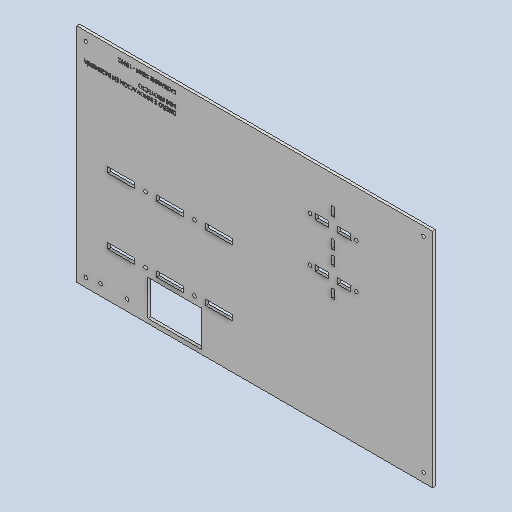
# Autodesk Inventor part: Base_proyecto
Saved by Autodesk Inventor 2022 (Build 260153000, 153)
## iProperties
Created: 2022-02-22
Part Number: Base_proyecto
Material: Generic
Document SubType Name: Modeling
Designer: katha
Density: 1 g/cm^3
Appearance: Default
Author: katha
Autodesk Inventor part; units mm, degrees
(part 1 of 2)
ref_plane "YZ Plane" through (0, 0, 0) normal (1, 0, 0) x (0, 1, 0)
ref_plane "XZ Plane" through (0, 0, 0) normal (0, 1, 0) x (-1, 0, 0)
ref_plane "XY Plane" through (0, 0, 0) normal (0, 0, 1) x (1, 0, 0)
sketch "Sketch1" plane through (0, 0, 0) normal (0, 0, 1) x (1, 0, 0)
  line L0 (200, 125) -> (-200, 125)
  line L1 (-200, 125) -> (-200, -125)
  line L2 (-200, -125) -> (200, -125)
  line L3 (200, -125) -> (200, 125)
  line L4 (200, 125) -> (-200, -125) construction
  line L5 (-200, 125) -> (200, -125) construction
  point P0 (0, 0)
  dimension "d0" = 400
  dimension "d1" = 250
  constraints: 12 end point, 2 midpoint, 2 parallel, 1 horizontal, 1 perpendicular
  measures "d0" distance of L2.end L1.end
  measures "d1" distance of L1.end L0.end
extrude "Extrusion1" add sketch "Sketch1" along normal blind 3.2
sketch "Sketch2" plane through (0, 0, 0) normal (0, 0, -1) x (-1, 0, 0)
  line L0 (-116.4, 20) -> (-116.4, 26.2) projected
  line L1 (-112.4, 26.2) -> (-112.4, 20) projected
  line L2 (-64.4, 20) -> (-64.4, 26.2) projected
  line L3 (-60.4, 26.2) -> (-60.4, 20) projected
  line L4 (-116.4, 70.2) -> (-116.4, 76.4) projected
  line L5 (-112.4, 76.4) -> (-112.4, 70.2) projected
  line L6 (-64.4, 70.2) -> (-64.4, 76.4) projected
  line L7 (-60.4, 76.4) -> (-60.4, 70.2) projected
  line L8 (-93.4, 76.4) -> (-108.4, 76.4) projected
  line L9 (-93.4, 70.2) -> (-108.4, 70.2) projected
  line L10 (-93.4, 76.4) -> (-93.4, 70.2) projected
  line L11 (-108.4, 76.4) -> (-108.4, 70.2) projected
  line L12 (-68.4, 76.4) -> (-83.4, 76.4) projected
  line L13 (-68.4, 70.2) -> (-83.4, 70.2) projected
  line L14 (-68.4, 76.4) -> (-68.4, 70.2) projected
  line L15 (-83.4, 76.4) -> (-83.4, 70.2) projected
  line L16 (-93.4, 26.2) -> (-108.4, 26.2) projected
  line L17 (-93.4, 20) -> (-108.4, 20) projected
  line L18 (-93.4, 26.2) -> (-93.4, 20) projected
  line L19 (-108.4, 26.2) -> (-108.4, 20) projected
  line L20 (-68.4, 26.2) -> (-83.4, 26.2) projected
  line L21 (-68.4, 20) -> (-83.4, 20) projected
  line L22 (-68.4, 26.2) -> (-68.4, 20) projected
  line L23 (-83.4, 26.2) -> (-83.4, 20) projected
  line L24 (69.5467, 5.2) -> (69.5467, -1) projected
  line L25 (25, 5.2) -> (55, 5.2) projected
  line L26 (80.0934, 5.2) -> (110.0934, 5.2) projected
  line L27 (124.6401, 5.2) -> (124.6401, -1) projected
  line L28 (135.1868, 5.2) -> (165.1868, 5.2) projected
  line L29 (55, -75) -> (25, -75) projected
  line L30 (110.0934, -75) -> (80.0934, -75) projected
  line L31 (165.1868, -75) -> (135.1868, -75) projected
  line L32 (124.6401, -68.8) -> (124.6401, -75) projected
  line L33 (69.5467, -68.8) -> (69.5467, -75) projected
  line L34 (-90, 35.2) -> (-90, 45.2) projected
  line L35 (-86.8, 45.2) -> (-86.8, 35.2) projected
  line L36 (-90, 35.2) -> (-86.8, 35.2) projected
  line L37 (-90, 45.2) -> (-86.8, 45.2) projected
  line L38 (-90, 51.2) -> (-86.8, 51.2) projected
  line L39 (-90, 51.2) -> (-90, 61.2) projected
  line L40 (-86.8, 61.2) -> (-86.8, 51.2) projected
  line L41 (-90, 61.2) -> (-86.8, 61.2) projected
  line L42 (165.1868, -1) -> (165.1868, 5.2) projected
  line L43 (165.1868, -1) -> (135.1868, -1) projected
  line L44 (135.1868, -1) -> (135.1868, 5.2) projected
  line L45 (120.6401, -1) -> (120.6401, 5.2) projected
  line L46 (124.6401, 5.2) -> (124.6401, -1) projected
  line L47 (65.5467, -1) -> (65.5467, 5.2) projected
  line L48 (120.6401, -75) -> (120.6401, -68.8) projected
  line L49 (135.1868, -75) -> (135.1868, -68.8) projected
  line L50 (135.1868, -68.8) -> (165.1868, -68.8) projected
  line L51 (165.1868, -75) -> (165.1868, -68.8) projected
  line L52 (80.0934, -68.8) -> (110.0934, -68.8) projected
  line L53 (80.0934, -75) -> (80.0934, -68.8) projected
  line L54 (110.0934, -75) -> (110.0934, -68.8) projected
  line L55 (25, -75) -> (25, -68.8) projected
  line L56 (25, -68.8) -> (55, -68.8) projected
  line L57 (55, -75) -> (55, -68.8) projected
  line L58 (65.5467, -75) -> (65.5467, -68.8) projected
  line L59 (55, -1) -> (25, -1) projected
  line L60 (25, -1) -> (25, 5.2) projected
  line L61 (55, -1) -> (55, 5.2) projected
  line L62 (80.0934, -1) -> (80.0934, 5.2) projected
  line L63 (110.0934, -1) -> (80.0934, -1) projected
  line L64 (110.0934, -1) -> (110.0934, 5.2) projected
  line L65 (55, -71.9) -> (135.1868, -71.9) construction
  line L66 (55, 2.1) -> (135.1868, 2.1) construction
  line L67 (64.0467, -68.8) -> (71.0467, -68.8) projected
  circle A0 centre (67.5467, -71.9) radius 2
  line L68 (95.0934, -68.8) -> (95.0934, -1) construction
  line L69 (95.0934, -34.9) -> (76.0096, -34.9) construction
  line L70 (67.5467, -68.8) -> (67.5467, -71.9) construction
  circle A1 centre (122.6401, -71.9) radius 2
  circle A2 centre (67.5467, 2.1) radius 2
  circle A3 centre (122.6401, 2.1) radius 2
  line L71 (-116.4, 23.1) -> (-112.4, 23.1) construction
  line L72 (-88.4, 45.2) -> (-88.4, 51.2) construction
  line L73 (-88.4, 48.2) -> (-97.8436, 48.2) construction
  circle A4 centre (-114.4, 23.1) radius 2
  circle A5 centre (-62.4, 23.1) radius 2
  circle A6 centre (-114.4, 73.3) radius 2
  circle A7 centre (-62.4, 73.3) radius 2
  line L74 (-90, 3.2) -> (-86.8, 3.2) projected
  line L75 (-90, 3.2) -> (-90, 13.2) projected
  line L76 (-86.8, 13.2) -> (-86.8, 3.2) projected
  line L77 (-90, 13.2) -> (-86.8, 13.2) projected
  line L78 (-90, 93.2) -> (-86.8, 93.2) projected
  line L79 (-90, 83.2) -> (-90, 93.2) projected
  line L80 (-86.8, 93.2) -> (-86.8, 83.2) projected
  line L81 (-90, 83.2) -> (-86.8, 83.2) projected
  line L82 (200, 125) -> (200, -125) projected
  point P0 (0, 0)
  dimension "d4" = 4
  dimension "d5" = 4
  constraints: 16 end point, 14 midpoint, 8 centre point, 6 symmetric about line, 2 horizontal, 1 point on line, 1 vertical, 6 other
  measures "d4" diameter of A0
  measures "d5" diameter of A4
extrude "Extrusion2" cut sketch "Sketch2" against normal blind 10 contours L10 L9 L11 L8 | L14 L13 L15 L12 | L18 L17 L19 L16 | L22 L21 L23 L20 | L25 L61 L59 L60 | L26 L64 L63 L62 | L28 L42 L43 L44 | L29 L55 L56 L57 | L30 L53 L52 L54 | L31 L49 L50 L51 | A0 | L34 L37 L35 L36 | L39 L41 L40 L38 | A1 | A2 | A3 | A4 | A5 | A6 | A7 | L75 L77 L76 L74 | L78 L80 L81 L79
sketch "Sketch3" plane through (0, 0, 3.2) normal (0, 0, 1) x (1, 0, 0)
  line L0 (-88.1097, 91.9364) -> (-249.5972, 91.9364) construction
  line L1 (-249.5972, 91.9364) -> (-249.5972, 106.9237) construction
  line L2 (-249.5972, 106.9237) -> (-88.1097, 106.9237) construction
  line L3 (-88.1097, 106.9237) -> (-88.1097, 91.9364) construction
  line L4 (-88.5956, 97.0895) -> (-88.5956, 93.0895)
  line L5 (-88.5956, 93.0895) -> (-89.4247, 93.0895)
  spline S0 degree 2 poles (-89.4247, 93.0895) (-90.3219, 93.0895) (-90.7267, 93.232) knots 0 0 0 1 1 1
  spline S1 degree 2 poles (-90.7267, 93.232) (-91.3097, 93.436) (-91.964, 94.4433) (-91.964, 95.1397) knots 0 0 0 1 2 2 2
  spline S2 degree 2 poles (-91.964, 95.1397) (-91.964, 95.7421) (-91.4458, 96.6555) (-90.6166, 97.0895) (-89.8684, 97.0895) knots 0 0 0 1 2 3 3 3
  line L6 (-89.8684, 97.0895) -> (-88.5956, 97.0895)
  line L7 (-88.9778, 96.7105) -> (-89.4409, 96.7105)
  spline S3 degree 2 poles (-89.4409, 96.7105) (-90.2701, 96.7105) (-90.5907, 96.6069) knots 0 0 0 1 1 1
  spline S4 degree 2 poles (-90.5907, 96.6069) (-91.0409, 96.4611) (-91.5591, 95.6967) (-91.5591, 95.1461) knots 0 0 0 1 2 2 2
  spline S5 degree 2 poles (-91.5591, 95.1461) (-91.5591, 94.5664) (-90.9988, 93.7469) (-90.4968, 93.5947) knots 0 0 0 1 2 2 2
  spline S6 degree 2 poles (-90.4968, 93.5947) (-90.1243, 93.4814) (-89.2595, 93.4814) knots 0 0 0 1 1 1
  line L8 (-89.2595, 93.4814) -> (-88.9778, 93.4814)
  line L9 (-88.9778, 93.4814) -> (-88.9778, 96.7105)
  line L10 (-92.683, 93.0895) -> (-93.0814, 93.0895)
  line L11 (-93.0814, 93.0895) -> (-93.0814, 97.0895)
  line L12 (-93.0814, 97.0895) -> (-92.683, 97.0895)
  line L13 (-92.683, 97.0895) -> (-92.683, 93.0895)
  line L14 (-93.5867, 96.3445) -> (-93.9267, 96.1405)
  spline S7 degree 2 poles (-93.9267, 96.1405) (-94.2863, 96.8012) (-94.7559, 96.8012) knots 0 0 0 1 1 1
  spline S8 degree 2 poles (-94.7559, 96.8012) (-94.9567, 96.8012) (-95.3097, 96.6133) (-95.4944, 96.2992) (-95.4944, 96.121) knots 0 0 0 1 2 3 3 3
  spline S9 degree 2 poles (-95.4944, 96.121) (-95.4944, 95.9202) (-95.3583, 95.7291) knots 0 0 0 1 1 1
  spline S10 degree 2 poles (-95.3583, 95.7291) (-95.1705, 95.4603) (-94.6749, 95.0846) knots 0 0 0 1 1 1
  spline S11 degree 2 poles (-94.6749, 95.0846) (-94.1729, 94.7089) (-94.0498, 94.5405) knots 0 0 0 1 1 1
  spline S12 degree 2 poles (-94.0498, 94.5405) (-93.8393, 94.2555) (-93.8393, 93.9283) knots 0 0 0 1 1 1
  spline S13 degree 2 poles (-93.8393, 93.9283) (-93.8393, 93.666) (-94.0887, 93.2352) (-94.5421, 92.9891) (-94.8077, 92.9891) knots 0 0 0 1 2 3 3 3
  spline S14 degree 2 poles (-94.8077, 92.9891) (-95.0927, 92.9891) (-95.5818, 93.2708) (-95.8571, 93.6465) knots 0 0 0 1 2 2 2
  line L15 (-95.8571, 93.6465) -> (-95.53, 93.8927)
  spline S15 degree 2 poles (-95.53, 93.8927) (-95.3065, 93.5947) (-94.9858, 93.4036) (-94.8012, 93.4036) knots 0 0 0 1 2 2 2
  spline S16 degree 2 poles (-94.8012, 93.4036) (-94.5583, 93.4036) (-94.2506, 93.6984) (-94.2506, 93.9121) knots 0 0 0 1 2 2 2
  spline S17 degree 2 poles (-94.2506, 93.9121) (-94.2506, 94.0417) (-94.3607, 94.2878) (-94.5033, 94.4303) knots 0 0 0 1 2 2 2
  spline S18 degree 2 poles (-94.5033, 94.4303) (-94.581, 94.5081) (-95.0215, 94.832) knots 0 0 0 1 1 1
  spline S19 degree 2 poles (-95.0215, 94.832) (-95.5397, 95.2142) (-95.9251, 95.8133) (-95.9251, 96.1146) knots 0 0 0 1 2 2 2
  spline S20 degree 2 poles (-95.9251, 96.1146) (-95.9251, 96.5486) (-95.2644, 97.1899) (-94.7915, 97.1899) knots 0 0 0 1 2 2 2
  spline S21 degree 2 poles (-94.7915, 97.1899) (-94.4288, 97.1899) (-93.8361, 96.8012) (-93.5867, 96.3445) knots 0 0 0 1 2 2 2
  line L16 (-96.7737, 93.0895) -> (-99.0668, 93.0895)
  line L17 (-99.0668, 93.0895) -> (-99.0668, 93.4814)
  line L18 (-99.0668, 93.4814) -> (-97.1721, 93.4814)
  line L19 (-97.1721, 93.4814) -> (-97.1721, 94.7348)
  line L20 (-97.1721, 94.7348) -> (-99.0506, 94.7348)
  line L21 (-99.0506, 94.7348) -> (-99.0506, 95.1267)
  line L22 (-99.0506, 95.1267) -> (-97.1721, 95.1267)
  line L23 (-97.1721, 95.1267) -> (-97.1721, 96.6976)
  line L24 (-97.1721, 96.6976) -> (-99.0506, 96.6976)
  line L25 (-99.0506, 96.6976) -> (-99.0506, 97.0895)
  line L26 (-99.0506, 97.0895) -> (-96.7737, 97.0895)
  line L27 (-96.7737, 97.0895) -> (-96.7737, 93.0895)
  line L28 (-99.7599, 97.0895) -> (-99.7599, 93.0895)
  line L29 (-99.7599, 93.0895) -> (-99.8474, 93.0895)
  line L30 (-99.8474, 93.0895) -> (-102.5097, 96.1534)
  line L31 (-102.5097, 96.1534) -> (-102.5097, 93.0895)
  line L32 (-102.5097, 93.0895) -> (-102.9049, 93.0895)
  line L33 (-102.9049, 93.0895) -> (-102.9049, 97.0895)
  line L34 (-102.9049, 97.0895) -> (-102.8142, 97.0895)
  line L35 (-102.8142, 97.0895) -> (-100.1745, 94.0611)
  line L36 (-100.1745, 94.0611) -> (-100.1745, 97.0895)
  line L37 (-100.1745, 97.0895) -> (-99.7599, 97.0895)
  line L38 (-102.1373, 92.2247) -> (-102.3284, 92.487)
  spline S22 degree 2 poles (-102.3284, 92.487) (-102.134, 92.6295) (-101.8652, 92.7299) (-101.713, 92.7299) knots 0 0 0 1 2 2 2
  spline S23 degree 2 poles (-101.713, 92.7299) (-101.5186, 92.7299) (-101.3114, 92.6295) knots 0 0 0 1 1 1
  spline S24 degree 2 poles (-101.3114, 92.6295) (-101.1365, 92.5421) (-101.0879, 92.5291) knots 0 0 0 1 1 1
  spline S25 degree 2 poles (-101.0879, 92.5291) (-101.0199, 92.5097) (-100.9454, 92.5097) knots 0 0 0 1 1 1
  spline S26 degree 2 poles (-100.9454, 92.5097) (-100.8514, 92.5097) (-100.6798, 92.5777) (-100.5146, 92.6976) knots 0 0 0 1 2 2 2
  line L39 (-100.5146, 92.6976) -> (-100.3365, 92.419)
  spline S27 degree 2 poles (-100.3365, 92.419) (-100.5826, 92.1534) (-100.9486, 92.1534) knots 0 0 0 1 1 1
  spline S28 degree 2 poles (-100.9486, 92.1534) (-101.1203, 92.1534) (-101.3632, 92.2635) knots 0 0 0 1 1 1
  spline S29 degree 2 poles (-101.3632, 92.2635) (-101.5931, 92.3737) (-101.7292, 92.3737) knots 0 0 0 1 1 1
  spline S30 degree 2 poles (-101.7292, 92.3737) (-101.8782, 92.3737) (-102.1373, 92.2247) knots 0 0 0 1 1 1
  spline S31 degree 2 poles (-105.7842, 92.9891) (-106.6911, 92.9891) (-107.9154, 94.2004) (-107.9154, 95.0878) knots 0 0 0 1 2 2 2
  spline S32 degree 2 poles (-107.9154, 95.0878) (-107.9154, 95.9656) (-106.6944, 97.1899) (-105.8166, 97.1899) knots 0 0 0 1 2 2 2
  spline S33 degree 2 poles (-105.8166, 97.1899) (-104.9259, 97.1899) (-103.7016, 95.972) (-103.7016, 95.1073) knots 0 0 0 1 2 2 2
  spline S34 degree 2 poles (-103.7016, 95.1073) (-103.7016, 94.5308) (-104.2587, 93.5461) (-105.2239, 92.9891) (-105.7842, 92.9891) knots 0 0 0 1 2 3 3 3
  spline S35 degree 2 poles (-105.8004, 93.3777) (-105.3567, 93.3777) (-104.5599, 93.8409) (-104.113, 94.6247) (-104.113, 95.1073) knots 0 0 0 1 2 3 3 3
  spline S36 degree 2 poles (-104.113, 95.1073) (-104.113, 95.8198) (-105.1041, 96.8012) (-105.8004, 96.8012) knots 0 0 0 1 2 2 2
  spline S37 degree 2 poles (-105.8004, 96.8012) (-106.2668, 96.8012) (-107.0603, 96.351) (-107.5041, 95.5672) (-107.5041, 95.0878) knots 0 0 0 1 2 3 3 3
  spline S38 degree 2 poles (-107.5041, 95.0878) (-107.5041, 94.6117) (-107.0603, 93.8409) (-106.2539, 93.3777) (-105.8004, 93.3777) knots 0 0 0 1 2 3 3 3
  line L40 (-110.2603, 93.0895) -> (-112.5535, 93.0895)
  line L41 (-112.5535, 93.0895) -> (-112.5535, 93.4814)
  line L42 (-112.5535, 93.4814) -> (-110.6587, 93.4814)
  line L43 (-110.6587, 93.4814) -> (-110.6587, 94.7348)
  line L44 (-110.6587, 94.7348) -> (-112.5373, 94.7348)
  line L45 (-112.5373, 94.7348) -> (-112.5373, 95.1267)
  line L46 (-112.5373, 95.1267) -> (-110.6587, 95.1267)
  line L47 (-110.6587, 95.1267) -> (-110.6587, 96.6976)
  line L48 (-110.6587, 96.6976) -> (-112.5373, 96.6976)
  line L49 (-112.5373, 96.6976) -> (-112.5373, 97.0895)
  line L50 (-112.5373, 97.0895) -> (-110.2603, 97.0895)
  line L51 (-110.2603, 97.0895) -> (-110.2603, 93.0895)
  line L52 (-114.73, 93.0895) -> (-115.1284, 93.0895)
  line L53 (-115.1284, 93.0895) -> (-115.1284, 97.0895)
  line L54 (-115.1284, 97.0895) -> (-114.73, 97.0895)
  line L55 (-114.73, 97.0895) -> (-114.73, 93.0895)
  line L56 (-116.0482, 97.0895) -> (-116.0482, 93.0895)
  line L57 (-116.0482, 93.0895) -> (-116.1356, 93.0895)
  line L58 (-116.1356, 93.0895) -> (-118.798, 96.1534)
  line L59 (-118.798, 96.1534) -> (-118.798, 93.0895)
  line L60 (-118.798, 93.0895) -> (-119.1931, 93.0895)
  line L61 (-119.1931, 93.0895) -> (-119.1931, 97.0895)
  line L62 (-119.1931, 97.0895) -> (-119.1024, 97.0895)
  line L63 (-119.1024, 97.0895) -> (-116.4628, 94.0611)
  line L64 (-116.4628, 94.0611) -> (-116.4628, 97.0895)
  line L65 (-116.4628, 97.0895) -> (-116.0482, 97.0895)
  line L66 (-120.168, 97.0895) -> (-120.168, 93.0895)
  line L67 (-120.168, 93.0895) -> (-120.2555, 93.0895)
  line L68 (-120.2555, 93.0895) -> (-122.9178, 96.1534)
  line L69 (-122.9178, 96.1534) -> (-122.9178, 93.0895)
  line L70 (-122.9178, 93.0895) -> (-123.313, 93.0895)
  line L71 (-123.313, 93.0895) -> (-123.313, 97.0895)
  line L72 (-123.313, 97.0895) -> (-123.2223, 97.0895)
  line L73 (-123.2223, 97.0895) -> (-120.5826, 94.0611)
  line L74 (-120.5826, 94.0611) -> (-120.5826, 97.0895)
  line L75 (-120.5826, 97.0895) -> (-120.168, 97.0895)
  spline S39 degree 2 poles (-126.1923, 92.9891) (-127.0992, 92.9891) (-128.3235, 94.2004) (-128.3235, 95.0878) knots 0 0 0 1 2 2 2
  spline S40 degree 2 poles (-128.3235, 95.0878) (-128.3235, 95.9656) (-127.1024, 97.1899) (-126.2247, 97.1899) knots 0 0 0 1 2 2 2
  spline S41 degree 2 poles (-126.2247, 97.1899) (-125.334, 97.1899) (-124.1097, 95.972) (-124.1097, 95.1073) knots 0 0 0 1 2 2 2
  spline S42 degree 2 poles (-124.1097, 95.1073) (-124.1097, 94.5308) (-124.6668, 93.5461) (-125.632, 92.9891) (-126.1923, 92.9891) knots 0 0 0 1 2 3 3 3
  spline S43 degree 2 poles (-126.2085, 93.3777) (-125.7648, 93.3777) (-124.968, 93.8409) (-124.5211, 94.6247) (-124.5211, 95.1073) knots 0 0 0 1 2 3 3 3
  spline S44 degree 2 poles (-124.5211, 95.1073) (-124.5211, 95.8198) (-125.5122, 96.8012) (-126.2085, 96.8012) knots 0 0 0 1 2 2 2
  spline S45 degree 2 poles (-126.2085, 96.8012) (-126.6749, 96.8012) (-127.4684, 96.351) (-127.9122, 95.5672) (-127.9122, 95.0878) knots 0 0 0 1 2 3 3 3
  spline S46 degree 2 poles (-127.9122, 95.0878) (-127.9122, 94.6117) (-127.4684, 93.8409) (-126.662, 93.3777) (-126.2085, 93.3777) knots 0 0 0 1 2 3 3 3
  line L76 (-128.819, 93.0895) -> (-129.2531, 93.0895)
  line L77 (-129.2531, 93.0895) -> (-130.581, 96.1826)
  line L78 (-130.581, 96.1826) -> (-131.9284, 93.0895)
  line L79 (-131.9284, 93.0895) -> (-132.3624, 93.0895)
  line L80 (-132.3624, 93.0895) -> (-130.6231, 97.0895)
  line L81 (-130.6231, 97.0895) -> (-130.5356, 97.0895)
  line L82 (-130.5356, 97.0895) -> (-128.819, 93.0895)
  line L83 (-134.6652, 93.0895) -> (-136.5308, 97.0895)
  line L84 (-136.5308, 97.0895) -> (-136.1, 97.0895)
  line L85 (-136.1, 97.0895) -> (-135.4717, 95.7712)
  line L86 (-135.4717, 95.7712) -> (-133.7486, 95.7712)
  line L87 (-133.7486, 95.7712) -> (-133.1267, 97.0895)
  line L88 (-133.1267, 97.0895) -> (-132.6798, 97.0895)
  line L89 (-132.6798, 97.0895) -> (-134.568, 93.0895)
  line L90 (-134.568, 93.0895) -> (-134.6652, 93.0895)
  line L91 (-134.6134, 93.938) -> (-133.93, 95.3858)
  line L92 (-133.93, 95.3858) -> (-135.2968, 95.3858)
  line L93 (-135.2968, 95.3858) -> (-134.6134, 93.938)
  line L94 (-140.8806, 93.8312) -> (-140.5664, 94.0741)
  spline S47 degree 2 poles (-140.5664, 94.0741) (-140.3041, 93.734) (-139.5721, 93.3842) (-139.1348, 93.3842) knots 0 0 0 1 2 2 2
  spline S48 degree 2 poles (-139.1348, 93.3842) (-138.6555, 93.3842) (-137.8393, 93.8441) (-137.3891, 94.6182) (-137.3891, 95.1008) knots 0 0 0 1 2 3 3 3
  spline S49 degree 2 poles (-137.3891, 95.1008) (-137.3891, 95.8328) (-138.3931, 96.8109) (-139.1575, 96.8109) knots 0 0 0 1 2 2 2
  spline S50 degree 2 poles (-139.1575, 96.8109) (-139.9996, 96.8109) (-140.5664, 96.1534) knots 0 0 0 1 1 1
  line L95 (-140.5664, 96.1534) -> (-140.8806, 96.3931)
  spline S51 degree 2 poles (-140.8806, 96.3931) (-140.5826, 96.772) (-139.6854, 97.1899) (-139.1348, 97.1899) knots 0 0 0 1 2 2 2
  spline S52 degree 2 poles (-139.1348, 97.1899) (-138.0822, 97.1899) (-137.4765, 96.4903) knots 0 0 0 1 1 1
  spline S53 degree 2 poles (-137.4765, 96.4903) (-136.968, 95.9008) (-136.968, 95.0652) knots 0 0 0 1 1 1
  spline S54 degree 2 poles (-136.968, 95.0652) (-136.968, 94.1874) (-138.202, 92.9891) (-139.1284, 92.9891) knots 0 0 0 1 2 2 2
  spline S55 degree 2 poles (-139.1284, 92.9891) (-139.6887, 92.9891) (-140.5923, 93.4328) (-140.8806, 93.8312) knots 0 0 0 1 2 2 2
  line L96 (-141.6255, 93.0895) -> (-142.0239, 93.0895)
  line L97 (-142.0239, 93.0895) -> (-142.0239, 97.0895)
  line L98 (-142.0239, 97.0895) -> (-141.6255, 97.0895)
  line L99 (-141.6255, 97.0895) -> (-141.6255, 93.0895)
  spline S56 degree 2 poles (-144.8482, 92.9891) (-145.7551, 92.9891) (-146.9794, 94.2004) (-146.9794, 95.0878) knots 0 0 0 1 2 2 2
  spline S57 degree 2 poles (-146.9794, 95.0878) (-146.9794, 95.9656) (-145.7583, 97.1899) (-144.8806, 97.1899) knots 0 0 0 1 2 2 2
  spline S58 degree 2 poles (-144.8806, 97.1899) (-143.9899, 97.1899) (-142.7656, 95.972) (-142.7656, 95.1073) knots 0 0 0 1 2 2 2
  spline S59 degree 2 poles (-142.7656, 95.1073) (-142.7656, 94.5308) (-143.3227, 93.5461) (-144.2879, 92.9891) (-144.8482, 92.9891) knots 0 0 0 1 2 3 3 3
  spline S60 degree 2 poles (-144.8644, 93.3777) (-144.4207, 93.3777) (-143.6239, 93.8409) (-143.1769, 94.6247) (-143.1769, 95.1073) knots 0 0 0 1 2 3 3 3
  spline S61 degree 2 poles (-143.1769, 95.1073) (-143.1769, 95.8198) (-144.168, 96.8012) (-144.8644, 96.8012) knots 0 0 0 1 2 2 2
  spline S62 degree 2 poles (-144.8644, 96.8012) (-145.3308, 96.8012) (-146.1243, 96.351) (-146.568, 95.5672) (-146.568, 95.0878) knots 0 0 0 1 2 3 3 3
  spline S63 degree 2 poles (-146.568, 95.0878) (-146.568, 94.6117) (-146.1243, 93.8409) (-145.3178, 93.3777) (-144.8644, 93.3777) knots 0 0 0 1 2 3 3 3
  line L100 (-145.062, 91.9364) -> (-145.645, 91.9364)
  line L101 (-145.645, 91.9364) -> (-144.845, 92.7753)
  line L102 (-144.845, 92.7753) -> (-144.4693, 92.7753)
  line L103 (-144.4693, 92.7753) -> (-145.062, 91.9364)
  line L104 (-147.7826, 97.0895) -> (-147.7826, 93.0895)
  line L105 (-147.7826, 93.0895) -> (-147.8701, 93.0895)
  line L106 (-147.8701, 93.0895) -> (-150.5324, 96.1534)
  line L107 (-150.5324, 96.1534) -> (-150.5324, 93.0895)
  line L108 (-150.5324, 93.0895) -> (-150.9275, 93.0895)
  line L109 (-150.9275, 93.0895) -> (-150.9275, 97.0895)
  line L110 (-150.9275, 97.0895) -> (-150.8369, 97.0895)
  line L111 (-150.8369, 97.0895) -> (-148.1972, 94.0611)
  line L112 (-148.1972, 94.0611) -> (-148.1972, 97.0895)
  line L113 (-148.1972, 97.0895) -> (-147.7826, 97.0895)
  line L114 (-153.4441, 93.0895) -> (-155.7373, 93.0895)
  line L115 (-155.7373, 93.0895) -> (-155.7373, 93.4814)
  line L116 (-155.7373, 93.4814) -> (-153.8425, 93.4814)
  line L117 (-153.8425, 93.4814) -> (-153.8425, 94.7348)
  line L118 (-153.8425, 94.7348) -> (-155.7211, 94.7348)
  line L119 (-155.7211, 94.7348) -> (-155.7211, 95.1267)
  line L120 (-155.7211, 95.1267) -> (-153.8425, 95.1267)
  line L121 (-153.8425, 95.1267) -> (-153.8425, 96.6976)
  line L122 (-153.8425, 96.6976) -> (-155.7211, 96.6976)
  line L123 (-155.7211, 96.6976) -> (-155.7211, 97.0895)
  line L124 (-155.7211, 97.0895) -> (-153.4441, 97.0895)
  line L125 (-153.4441, 97.0895) -> (-153.4441, 93.0895)
  line L126 (-156.4304, 97.0895) -> (-156.4304, 93.0895)
  line L127 (-156.4304, 93.0895) -> (-156.5178, 93.0895)
  line L128 (-156.5178, 93.0895) -> (-159.1802, 96.1534)
  line L129 (-159.1802, 96.1534) -> (-159.1802, 93.0895)
  line L130 (-159.1802, 93.0895) -> (-159.5753, 93.0895)
  line L131 (-159.5753, 93.0895) -> (-159.5753, 97.0895)
  line L132 (-159.5753, 97.0895) -> (-159.4846, 97.0895)
  line L133 (-159.4846, 97.0895) -> (-156.845, 94.0611)
  line L134 (-156.845, 94.0611) -> (-156.845, 97.0895)
  line L135 (-156.845, 97.0895) -> (-156.4304, 97.0895)
  line L136 (-162.0336, 93.0895) -> (-162.432, 93.0895)
  line L137 (-162.432, 93.0895) -> (-162.432, 97.0895)
  line L138 (-162.432, 97.0895) -> (-162.0336, 97.0895)
  line L139 (-162.0336, 97.0895) -> (-162.0336, 93.0895)
  line L140 (-163.3518, 97.0895) -> (-163.3518, 93.0895)
  line L141 (-163.3518, 93.0895) -> (-163.4393, 93.0895)
  line L142 (-163.4393, 93.0895) -> (-166.1016, 96.1534)
  line L143 (-166.1016, 96.1534) -> (-166.1016, 93.0895)
  line L144 (-166.1016, 93.0895) -> (-166.4968, 93.0895)
  line L145 (-166.4968, 93.0895) -> (-166.4968, 97.0895)
  line L146 (-166.4968, 97.0895) -> (-166.4061, 97.0895)
  line L147 (-166.4061, 97.0895) -> (-163.7664, 94.0611)
  line L148 (-163.7664, 94.0611) -> (-163.7664, 97.0895)
  line L149 (-163.7664, 97.0895) -> (-163.3518, 97.0895)
  line L150 (-171.3259, 93.7599) -> (-171.015, 94.0546)
  spline S64 degree 2 poles (-171.015, 94.0546) (-170.6814, 93.7275) (-169.8846, 93.3874) (-169.5057, 93.3874) knots 0 0 0 1 2 2 2
  spline S65 degree 2 poles (-169.5057, 93.3874) (-169.0361, 93.3874) (-168.1842, 93.8506) (-167.7178, 94.6409) (-167.7178, 95.0814) knots 0 0 0 1 2 3 3 3
  spline S66 degree 2 poles (-167.7178, 95.0814) (-167.7178, 95.5316) (-168.2037, 96.3445) (-169.0555, 96.8077) (-169.564, 96.8077) knots 0 0 0 1 2 3 3 3
  spline S67 degree 2 poles (-169.564, 96.8077) (-170.1826, 96.8077) (-171.0377, 96.1113) (-171.1154, 95.5575) knots 0 0 0 1 2 2 2
  line L151 (-171.1154, 95.5575) -> (-169.8393, 95.5575)
  line L152 (-169.8393, 95.5575) -> (-169.8393, 95.172)
  line L153 (-169.8393, 95.172) -> (-171.5624, 95.172)
  spline S68 degree 2 poles (-171.5624, 95.172) (-171.5559, 96.0984) (-170.4676, 97.1899) (-169.5543, 97.1899) knots 0 0 0 1 2 2 2
  spline S69 degree 2 poles (-169.5543, 97.1899) (-168.4433, 97.1899) (-167.7988, 96.4352) knots 0 0 0 1 1 1
  spline S70 degree 2 poles (-167.7988, 96.4352) (-167.3, 95.8522) (-167.3, 95.0878) knots 0 0 0 1 1 1
  spline S71 degree 2 poles (-167.3, 95.0878) (-167.3, 94.521) (-167.8701, 93.5397) (-168.8644, 92.9891) (-169.4927, 92.9891) knots 0 0 0 1 2 3 3 3
  spline S72 degree 2 poles (-169.4927, 92.9891) (-170.0012, 92.9891) (-170.8984, 93.355) (-171.3259, 93.7599) knots 0 0 0 1 2 2 2
  line L154 (-172.3267, 93.0895) -> (-174.6199, 93.0895)
  line L155 (-174.6199, 93.0895) -> (-174.6199, 93.4814)
  line L156 (-174.6199, 93.4814) -> (-172.7251, 93.4814)
  line L157 (-172.7251, 93.4814) -> (-172.7251, 94.7348)
  line L158 (-172.7251, 94.7348) -> (-174.6037, 94.7348)
  line L159 (-174.6037, 94.7348) -> (-174.6037, 95.1267)
  line L160 (-174.6037, 95.1267) -> (-172.7251, 95.1267)
  line L161 (-172.7251, 95.1267) -> (-172.7251, 96.6976)
  line L162 (-172.7251, 96.6976) -> (-174.6037, 96.6976)
  line L163 (-174.6037, 96.6976) -> (-174.6037, 97.0895)
  line L164 (-174.6037, 97.0895) -> (-172.3267, 97.0895)
  line L165 (-172.3267, 97.0895) -> (-172.3267, 93.0895)
  line L166 (-175.313, 97.0895) -> (-175.313, 93.0895)
  line L167 (-175.313, 93.0895) -> (-175.4004, 93.0895)
  line L168 (-175.4004, 93.0895) -> (-178.0628, 96.1534)
  line L169 (-178.0628, 96.1534) -> (-178.0628, 93.0895)
  line L170 (-178.0628, 93.0895) -> (-178.4579, 93.0895)
  line L171 (-178.4579, 93.0895) -> (-178.4579, 97.0895)
  line L172 (-178.4579, 97.0895) -> (-178.3672, 97.0895)
  line L173 (-178.3672, 97.0895) -> (-175.7276, 94.0611)
  line L174 (-175.7276, 94.0611) -> (-175.7276, 97.0895)
  line L175 (-175.7276, 97.0895) -> (-175.313, 97.0895)
  line L176 (-179.3745, 93.0895) -> (-179.7729, 93.0895)
  line L177 (-179.7729, 93.0895) -> (-179.7729, 97.0895)
  line L178 (-179.7729, 97.0895) -> (-179.3745, 97.0895)
  line L179 (-179.3745, 97.0895) -> (-179.3745, 93.0895)
  line L180 (-180.6927, 93.0895) -> (-182.9858, 93.0895)
  line L181 (-182.9858, 93.0895) -> (-182.9858, 93.4814)
  line L182 (-182.9858, 93.4814) -> (-181.0911, 93.4814)
  line L183 (-181.0911, 93.4814) -> (-181.0911, 94.7348)
  line L184 (-181.0911, 94.7348) -> (-182.9697, 94.7348)
  line L185 (-182.9697, 94.7348) -> (-182.9697, 95.1267)
  line L186 (-182.9697, 95.1267) -> (-181.0911, 95.1267)
  line L187 (-181.0911, 95.1267) -> (-181.0911, 96.6976)
  line L188 (-181.0911, 96.6976) -> (-182.9697, 96.6976)
  line L189 (-182.9697, 96.6976) -> (-182.9697, 97.0895)
  line L190 (-182.9697, 97.0895) -> (-180.6927, 97.0895)
  line L191 (-180.6927, 97.0895) -> (-180.6927, 93.0895)
  line L192 (-183.6984, 93.0895) -> (-184.4952, 93.0895)
  spline S73 degree 2 poles (-184.4952, 93.0895) (-185.1591, 93.0895) (-185.3956, 93.1445) knots 0 0 0 1 1 1
  spline S74 degree 2 poles (-185.3956, 93.1445) (-185.7518, 93.2255) (-186.1956, 93.7631) (-186.1956, 94.155) knots 0 0 0 1 2 2 2
  spline S75 degree 2 poles (-186.1956, 94.155) (-186.1956, 94.4822) (-185.8879, 94.9777) (-185.3178, 95.2303) (-184.8158, 95.2336) knots 0 0 0 1 2 3 3 3
  line L193 (-184.8158, 95.2336) -> (-186.2539, 97.0895)
  line L194 (-186.2539, 97.0895) -> (-185.7583, 97.0895)
  line L195 (-185.7583, 97.0895) -> (-184.3235, 95.2336)
  line L196 (-184.3235, 95.2336) -> (-184.0968, 95.2336)
  line L197 (-184.0968, 95.2336) -> (-184.0968, 97.0895)
  line L198 (-184.0968, 97.0895) -> (-183.6984, 97.0895)
  line L199 (-183.6984, 97.0895) -> (-183.6984, 93.0895)
  line L200 (-184.0968, 93.4814) -> (-184.0968, 94.8417)
  line L201 (-184.0968, 94.8417) -> (-184.7867, 94.8482)
  spline S76 degree 2 poles (-184.7867, 94.8482) (-185.185, 94.8482) (-185.5705, 94.6959) (-185.7842, 94.3591) (-185.7842, 94.1518) knots 0 0 0 1 2 3 3 3
  spline S77 degree 2 poles (-185.7842, 94.1518) (-185.7842, 93.951) (-185.5672, 93.6239) (-185.2142, 93.4814) (-184.8029, 93.4814) knots 0 0 0 1 2 3 3 3
  line L202 (-184.8029, 93.4814) -> (-184.0968, 93.4814)
  line L203 (-186.9988, 93.0895) -> (-187.3972, 93.0895)
  line L204 (-187.3972, 93.0895) -> (-187.3972, 97.0895)
  line L205 (-187.3972, 97.0895) -> (-186.9988, 97.0895)
  line L206 (-186.9988, 97.0895) -> (-186.9988, 93.0895)
  line L207 (-187.3842, 91.9364) -> (-187.9672, 91.9364)
  line L208 (-187.9672, 91.9364) -> (-187.1672, 92.7753)
  line L209 (-187.1672, 92.7753) -> (-186.7915, 92.7753)
  line L210 (-186.7915, 92.7753) -> (-187.3842, 91.9364)
  line L211 (-189.9462, 93.0895) -> (-191.8118, 97.0895)
  line L212 (-191.8118, 97.0895) -> (-191.381, 97.0895)
  line L213 (-191.381, 97.0895) -> (-190.7527, 95.7712)
  line L214 (-190.7527, 95.7712) -> (-189.0296, 95.7712)
  line L215 (-189.0296, 95.7712) -> (-188.4077, 97.0895)
  line L216 (-188.4077, 97.0895) -> (-187.9607, 97.0895)
  line L217 (-187.9607, 97.0895) -> (-189.849, 93.0895)
  line L218 (-189.849, 93.0895) -> (-189.9462, 93.0895)
  line L219 (-189.8944, 93.938) -> (-189.211, 95.3858)
  line L220 (-189.211, 95.3858) -> (-190.5778, 95.3858)
  line L221 (-190.5778, 95.3858) -> (-189.8944, 93.938)
  line L222 (-88.4142, 103.8802) -> (-88.981, 99.8802)
  line L223 (-88.981, 99.8802) -> (-89.049, 99.8802)
  line L224 (-89.049, 99.8802) -> (-90.6749, 103.1612)
  line L225 (-90.6749, 103.1612) -> (-92.2879, 99.8802)
  line L226 (-92.2879, 99.8802) -> (-92.3494, 99.8802)
  line L227 (-92.3494, 99.8802) -> (-92.9227, 103.8802)
  line L228 (-92.9227, 103.8802) -> (-92.5308, 103.8802)
  line L229 (-92.5308, 103.8802) -> (-92.1389, 101.0203)
  line L230 (-92.1389, 101.0203) -> (-90.7203, 103.8802)
  line L231 (-90.7203, 103.8802) -> (-90.6166, 103.8802)
  line L232 (-90.6166, 103.8802) -> (-89.1915, 100.9976)
  line L233 (-89.1915, 100.9976) -> (-88.7996, 103.8802)
  line L234 (-88.7996, 103.8802) -> (-88.4142, 103.8802)
  line L235 (-93.6579, 99.8802) -> (-94.0563, 99.8802)
  line L236 (-94.0563, 99.8802) -> (-94.0563, 103.8802)
  line L237 (-94.0563, 103.8802) -> (-93.6579, 103.8802)
  line L238 (-93.6579, 103.8802) -> (-93.6579, 99.8802)
  line L239 (-94.9761, 103.8802) -> (-94.9761, 99.8802)
  line L240 (-94.9761, 99.8802) -> (-95.0636, 99.8802)
  line L241 (-95.0636, 99.8802) -> (-97.7259, 102.9442)
  line L242 (-97.7259, 102.9442) -> (-97.7259, 99.8802)
  line L243 (-97.7259, 99.8802) -> (-98.1211, 99.8802)
  line L244 (-98.1211, 99.8802) -> (-98.1211, 103.8802)
  line L245 (-98.1211, 103.8802) -> (-98.0304, 103.8802)
  line L246 (-98.0304, 103.8802) -> (-95.3907, 100.8519)
  line L247 (-95.3907, 100.8519) -> (-95.3907, 103.8802)
  line L248 (-95.3907, 103.8802) -> (-94.9761, 103.8802)
  line L249 (-99.0377, 99.8802) -> (-99.4361, 99.8802)
  line L250 (-99.4361, 99.8802) -> (-99.4361, 103.8802)
  line L251 (-99.4361, 103.8802) -> (-99.0377, 103.8802)
  line L252 (-99.0377, 103.8802) -> (-99.0377, 99.8802)
  line L253 (-101.8911, 99.8802) -> (-102.6879, 99.8802)
  spline S78 degree 2 poles (-102.6879, 99.8802) (-103.3713, 99.8802) (-103.6109, 99.9385) knots 0 0 0 1 1 1
  spline S79 degree 2 poles (-103.6109, 99.9385) (-103.9543, 100.026) (-104.3883, 100.5506) (-104.3883, 100.9458) knots 0 0 0 1 2 2 2
  spline S80 degree 2 poles (-104.3883, 100.9458) (-104.3883, 101.3474) (-103.964, 101.8656) (-103.5915, 101.9563) knots 0 0 0 1 2 2 2
  spline S81 degree 2 poles (-103.5915, 101.9563) (-103.3195, 102.0211) (-102.5745, 102.0211) knots 0 0 0 1 1 1
  line L254 (-102.5745, 102.0211) -> (-102.2895, 102.0211)
  line L255 (-102.2895, 102.0211) -> (-102.2895, 103.8802)
  line L256 (-102.2895, 103.8802) -> (-101.8911, 103.8802)
  line L257 (-101.8911, 103.8802) -> (-101.8911, 99.8802)
  line L258 (-102.2895, 100.2721) -> (-102.2895, 101.6292)
  line L259 (-102.2895, 101.6292) -> (-102.9664, 101.6389)
  spline S82 degree 2 poles (-102.9664, 101.6389) (-103.3778, 101.6389) (-103.7599, 101.4867) (-103.9769, 101.1531) (-103.9769, 100.949) knots 0 0 0 1 2 3 3 3
  spline S83 degree 2 poles (-103.9769, 100.949) (-103.9769, 100.7482) (-103.7599, 100.4146) (-103.4037, 100.2721) (-102.9956, 100.2721) knots 0 0 0 1 2 3 3 3
  line L260 (-102.9956, 100.2721) -> (-102.2895, 100.2721)
  line L261 (-105.2109, 99.8802) -> (-106.0077, 99.8802)
  spline S84 degree 2 poles (-106.0077, 99.8802) (-106.6717, 99.8802) (-106.9081, 99.9353) knots 0 0 0 1 1 1
  spline S85 degree 2 poles (-106.9081, 99.9353) (-107.2644, 100.0162) (-107.7081, 100.5539) (-107.7081, 100.9458) knots 0 0 0 1 2 2 2
  spline S86 degree 2 poles (-107.7081, 100.9458) (-107.7081, 101.2729) (-107.4004, 101.7685) (-106.8304, 102.0211) (-106.3284, 102.0243) knots 0 0 0 1 2 3 3 3
  line L262 (-106.3284, 102.0243) -> (-107.7664, 103.8802)
  line L263 (-107.7664, 103.8802) -> (-107.2709, 103.8802)
  line L264 (-107.2709, 103.8802) -> (-105.8361, 102.0243)
  line L265 (-105.8361, 102.0243) -> (-105.6093, 102.0243)
  line L266 (-105.6093, 102.0243) -> (-105.6093, 103.8802)
  line L267 (-105.6093, 103.8802) -> (-105.2109, 103.8802)
  line L268 (-105.2109, 103.8802) -> (-105.2109, 99.8802)
  line L269 (-105.6093, 100.2721) -> (-105.6093, 101.6324)
  line L270 (-105.6093, 101.6324) -> (-106.2992, 101.6389)
  spline S87 degree 2 poles (-106.2992, 101.6389) (-106.6976, 101.6389) (-107.083, 101.4867) (-107.2968, 101.1498) (-107.2968, 100.9426) knots 0 0 0 1 2 3 3 3
  spline S88 degree 2 poles (-107.2968, 100.9426) (-107.2968, 100.7417) (-107.0798, 100.4146) (-106.7267, 100.2721) (-106.3154, 100.2721) knots 0 0 0 1 2 3 3 3
  line L271 (-106.3154, 100.2721) -> (-105.6093, 100.2721)
  spline S89 degree 2 poles (-110.4741, 99.7798) (-111.381, 99.7798) (-112.6053, 100.9911) (-112.6053, 101.8786) knots 0 0 0 1 2 2 2
  spline S90 degree 2 poles (-112.6053, 101.8786) (-112.6053, 102.7563) (-111.3842, 103.9806) (-110.5065, 103.9806) knots 0 0 0 1 2 2 2
  spline S91 degree 2 poles (-110.5065, 103.9806) (-109.6158, 103.9806) (-108.3915, 102.7628) (-108.3915, 101.898) knots 0 0 0 1 2 2 2
  spline S92 degree 2 poles (-108.3915, 101.898) (-108.3915, 101.3215) (-108.9486, 100.3369) (-109.9138, 99.7798) (-110.4741, 99.7798) knots 0 0 0 1 2 3 3 3
  spline S93 degree 2 poles (-110.4903, 100.1685) (-110.0466, 100.1685) (-109.2498, 100.6316) (-108.8029, 101.4154) (-108.8029, 101.898) knots 0 0 0 1 2 3 3 3
  spline S94 degree 2 poles (-108.8029, 101.898) (-108.8029, 102.6106) (-109.7939, 103.5919) (-110.4903, 103.5919) knots 0 0 0 1 2 2 2
  spline S95 degree 2 poles (-110.4903, 103.5919) (-110.9567, 103.5919) (-111.7502, 103.1417) (-112.1939, 102.3579) (-112.1939, 101.8786) knots 0 0 0 1 2 3 3 3
  spline S96 degree 2 poles (-112.1939, 101.8786) (-112.1939, 101.4025) (-111.7502, 100.6316) (-110.9437, 100.1685) (-110.4903, 100.1685) knots 0 0 0 1 2 3 3 3
  line L272 (-113.0911, 99.8802) -> (-113.551, 99.8802)
  line L273 (-113.551, 99.8802) -> (-114.5778, 101.5385)
  line L274 (-114.5778, 101.5385) -> (-115.5883, 99.8802)
  line L275 (-115.5883, 99.8802) -> (-116.045, 99.8802)
  line L276 (-116.045, 99.8802) -> (-114.7786, 101.9693)
  line L277 (-114.7786, 101.9693) -> (-114.7786, 103.8802)
  line L278 (-114.7786, 103.8802) -> (-114.3834, 103.8802)
  line L279 (-114.3834, 103.8802) -> (-114.3834, 101.9693)
  line L280 (-114.3834, 101.9693) -> (-113.0911, 99.8802)
  line L281 (-116.7024, 99.8802) -> (-118.9956, 99.8802)
  line L282 (-118.9956, 99.8802) -> (-118.9956, 100.2721)
  line L283 (-118.9956, 100.2721) -> (-117.1008, 100.2721)
  line L284 (-117.1008, 100.2721) -> (-117.1008, 101.5255)
  line L285 (-117.1008, 101.5255) -> (-118.9794, 101.5255)
  line L286 (-118.9794, 101.5255) -> (-118.9794, 101.9175)
  line L287 (-118.9794, 101.9175) -> (-117.1008, 101.9175)
  line L288 (-117.1008, 101.9175) -> (-117.1008, 103.4883)
  line L289 (-117.1008, 103.4883) -> (-118.9794, 103.4883)
  line L290 (-118.9794, 103.4883) -> (-118.9794, 103.8802)
  line L291 (-118.9794, 103.8802) -> (-116.7024, 103.8802)
  line L292 (-116.7024, 103.8802) -> (-116.7024, 99.8802)
  line L293 (-123.4134, 100.6219) -> (-123.0992, 100.8648)
  spline S97 degree 2 poles (-123.0992, 100.8648) (-122.8369, 100.5247) (-122.1049, 100.1749) (-121.6676, 100.1749) knots 0 0 0 1 2 2 2
  spline S98 degree 2 poles (-121.6676, 100.1749) (-121.1883, 100.1749) (-120.3721, 100.6349) (-119.9219, 101.4089) (-119.9219, 101.8915) knots 0 0 0 1 2 3 3 3
  spline S99 degree 2 poles (-119.9219, 101.8915) (-119.9219, 102.6235) (-120.9259, 103.6017) (-121.6903, 103.6017) knots 0 0 0 1 2 2 2
  spline S100 degree 2 poles (-121.6903, 103.6017) (-122.5324, 103.6017) (-123.0992, 102.9442) knots 0 0 0 1 1 1
  line L294 (-123.0992, 102.9442) -> (-123.4134, 103.1838)
  spline S101 degree 2 poles (-123.4134, 103.1838) (-123.1154, 103.5628) (-122.2182, 103.9806) (-121.6676, 103.9806) knots 0 0 0 1 2 2 2
  spline S102 degree 2 poles (-121.6676, 103.9806) (-120.615, 103.9806) (-120.0093, 103.281) knots 0 0 0 1 1 1
  spline S103 degree 2 poles (-120.0093, 103.281) (-119.5008, 102.6915) (-119.5008, 101.8559) knots 0 0 0 1 1 1
  spline S104 degree 2 poles (-119.5008, 101.8559) (-119.5008, 100.9782) (-120.7348, 99.7798) (-121.6612, 99.7798) knots 0 0 0 1 2 2 2
  spline S105 degree 2 poles (-121.6612, 99.7798) (-122.2215, 99.7798) (-123.1251, 100.2235) (-123.4134, 100.6219) knots 0 0 0 1 2 2 2
  line L295 (-123.8182, 100.2721) -> (-123.8182, 99.8802)
  line L296 (-123.8182, 99.8802) -> (-126.0077, 99.8802)
  line L297 (-126.0077, 99.8802) -> (-126.0077, 100.2721)
  line L298 (-126.0077, 100.2721) -> (-125.117, 100.2721)
  line L299 (-125.117, 100.2721) -> (-125.117, 103.8802)
  line L300 (-125.117, 103.8802) -> (-124.7089, 103.8802)
  line L301 (-124.7089, 103.8802) -> (-124.7089, 100.2721)
  line L302 (-124.7089, 100.2721) -> (-123.8182, 100.2721)
  spline S106 degree 2 poles (-128.4919, 99.7798) (-129.3988, 99.7798) (-130.6231, 100.9911) (-130.6231, 101.8786) knots 0 0 0 1 2 2 2
  spline S107 degree 2 poles (-130.6231, 101.8786) (-130.6231, 102.7563) (-129.402, 103.9806) (-128.5243, 103.9806) knots 0 0 0 1 2 2 2
  spline S108 degree 2 poles (-128.5243, 103.9806) (-127.6336, 103.9806) (-126.4093, 102.7628) (-126.4093, 101.898) knots 0 0 0 1 2 2 2
  spline S109 degree 2 poles (-126.4093, 101.898) (-126.4093, 101.3215) (-126.9664, 100.3369) (-127.9316, 99.7798) (-128.4919, 99.7798) knots 0 0 0 1 2 3 3 3
  spline S110 degree 2 poles (-128.5081, 100.1685) (-128.0644, 100.1685) (-127.2676, 100.6316) (-126.8207, 101.4154) (-126.8207, 101.898) knots 0 0 0 1 2 3 3 3
  spline S111 degree 2 poles (-126.8207, 101.898) (-126.8207, 102.6106) (-127.8118, 103.5919) (-128.5081, 103.5919) knots 0 0 0 1 2 2 2
  spline S112 degree 2 poles (-128.5081, 103.5919) (-128.9745, 103.5919) (-129.768, 103.1417) (-130.2118, 102.3579) (-130.2118, 101.8786) knots 0 0 0 1 2 3 3 3
  spline S113 degree 2 poles (-130.2118, 101.8786) (-130.2118, 101.4025) (-129.768, 100.6316) (-128.9616, 100.1685) (-128.5081, 100.1685) knots 0 0 0 1 2 3 3 3
  line L303 (-88.5956, 113.4617) -> (-89.0037, 113.4617)
  line L304 (-89.0037, 113.4617) -> (-89.0037, 114.9613)
  line L305 (-89.0037, 114.9613) -> (-90.6037, 113.4617)
  line L306 (-90.6037, 113.4617) -> (-91.1446, 113.4617)
  line L307 (-91.1446, 113.4617) -> (-89.2174, 115.256)
  line L308 (-89.2174, 115.256) -> (-91.2935, 117.4617)
  line L309 (-91.2935, 117.4617) -> (-90.7559, 117.4617)
  line L310 (-90.7559, 117.4617) -> (-89.0037, 115.5993)
  line L311 (-89.0037, 115.5993) -> (-89.0037, 117.4617)
  line L312 (-89.0037, 117.4617) -> (-88.5956, 117.4617)
  line L313 (-88.5956, 117.4617) -> (-88.5956, 113.4617)
  line L314 (-93.5186, 113.4617) -> (-95.3842, 117.4617)
  line L315 (-95.3842, 117.4617) -> (-94.9535, 117.4617)
  line L316 (-94.9535, 117.4617) -> (-94.3251, 116.1435)
  line L317 (-94.3251, 116.1435) -> (-92.602, 116.1435)
  line L318 (-92.602, 116.1435) -> (-91.9802, 117.4617)
  line L319 (-91.9802, 117.4617) -> (-91.5332, 117.4617)
  line L320 (-91.5332, 117.4617) -> (-93.4215, 113.4617)
  line L321 (-93.4215, 113.4617) -> (-93.5186, 113.4617)
  line L322 (-93.4668, 114.3103) -> (-92.7834, 115.7581)
  line L323 (-92.7834, 115.7581) -> (-94.1502, 115.7581)
  line L324 (-94.1502, 115.7581) -> (-93.4668, 114.3103)
  line L325 (-95.6109, 113.8536) -> (-95.6109, 113.4617)
  line L326 (-95.6109, 113.4617) -> (-97.8004, 113.4617)
  line L327 (-97.8004, 113.4617) -> (-97.8004, 113.8536)
  line L328 (-97.8004, 113.8536) -> (-96.9097, 113.8536)
  line L329 (-96.9097, 113.8536) -> (-96.9097, 117.4617)
  line L330 (-96.9097, 117.4617) -> (-96.5016, 117.4617)
  line L331 (-96.5016, 117.4617) -> (-96.5016, 113.8536)
  line L332 (-96.5016, 113.8536) -> (-95.6109, 113.8536)
  line L333 (-98.3737, 113.4617) -> (-98.7721, 113.4617)
  line L334 (-98.7721, 113.4617) -> (-98.7721, 115.1394)
  line L335 (-98.7721, 115.1394) -> (-100.8093, 115.1394)
  line L336 (-100.8093, 115.1394) -> (-100.8093, 113.4617)
  line L337 (-100.8093, 113.4617) -> (-101.2077, 113.4617)
  line L338 (-101.2077, 113.4617) -> (-101.2077, 117.4617)
  line L339 (-101.2077, 117.4617) -> (-100.8093, 117.4617)
  line L340 (-100.8093, 117.4617) -> (-100.8093, 115.5313)
  line L341 (-100.8093, 115.5313) -> (-98.7721, 115.5313)
  line L342 (-98.7721, 115.5313) -> (-98.7721, 117.4617)
  line L343 (-98.7721, 117.4617) -> (-98.3737, 117.4617)
  line L344 (-98.3737, 117.4617) -> (-98.3737, 113.4617)
  line L345 (-103.8118, 113.4617) -> (-105.6773, 117.4617)
  line L346 (-105.6773, 117.4617) -> (-105.2466, 117.4617)
  line L347 (-105.2466, 117.4617) -> (-104.6182, 116.1435)
  line L348 (-104.6182, 116.1435) -> (-102.8952, 116.1435)
  line L349 (-102.8952, 116.1435) -> (-102.2733, 117.4617)
  line L350 (-102.2733, 117.4617) -> (-101.8263, 117.4617)
  line L351 (-101.8263, 117.4617) -> (-103.7146, 113.4617)
  line L352 (-103.7146, 113.4617) -> (-103.8118, 113.4617)
  line L353 (-103.7599, 114.3103) -> (-103.0765, 115.7581)
  line L354 (-103.0765, 115.7581) -> (-104.4433, 115.7581)
  line L355 (-104.4433, 115.7581) -> (-103.7599, 114.3103)
  line L356 (-106.3219, 113.4617) -> (-107.1186, 113.4617)
  spline S114 degree 2 poles (-107.1186, 113.4617) (-107.7826, 113.4617) (-108.019, 113.5168) knots 0 0 0 1 1 1
  spline S115 degree 2 poles (-108.019, 113.5168) (-108.3753, 113.5977) (-108.819, 114.1354) (-108.819, 114.5273) knots 0 0 0 1 2 2 2
  spline S116 degree 2 poles (-108.819, 114.5273) (-108.819, 114.8544) (-108.5114, 115.35) (-107.9413, 115.6026) (-107.4393, 115.6058) knots 0 0 0 1 2 3 3 3
  line L357 (-107.4393, 115.6058) -> (-108.8773, 117.4617)
  line L358 (-108.8773, 117.4617) -> (-108.3818, 117.4617)
  line L359 (-108.3818, 117.4617) -> (-106.947, 115.6058)
  line L360 (-106.947, 115.6058) -> (-106.7203, 115.6058)
  line L361 (-106.7203, 115.6058) -> (-106.7203, 117.4617)
  line L362 (-106.7203, 117.4617) -> (-106.3219, 117.4617)
  line L363 (-106.3219, 117.4617) -> (-106.3219, 113.4617)
  line L364 (-106.7203, 113.8536) -> (-106.7203, 115.2139)
  line L365 (-106.7203, 115.2139) -> (-107.4101, 115.2204)
  spline S117 degree 2 poles (-107.4101, 115.2204) (-107.8085, 115.2204) (-108.1939, 115.0682) (-108.4077, 114.7313) (-108.4077, 114.524) knots 0 0 0 1 2 3 3 3
  spline S118 degree 2 poles (-108.4077, 114.524) (-108.4077, 114.3232) (-108.1907, 113.9961) (-107.8377, 113.8536) (-107.4263, 113.8536) knots 0 0 0 1 2 3 3 3
  line L366 (-107.4263, 113.8536) -> (-106.7203, 113.8536)
  line L367 (-109.6223, 113.4617) -> (-110.0207, 113.4617)
  line L368 (-110.0207, 113.4617) -> (-110.0207, 117.4617)
  line L369 (-110.0207, 117.4617) -> (-109.6223, 117.4617)
  line L370 (-109.6223, 117.4617) -> (-109.6223, 113.4617)
  line L371 (-110.9405, 117.4617) -> (-110.9405, 113.4617)
  line L372 (-110.9405, 113.4617) -> (-111.028, 113.4617)
  line L373 (-111.028, 113.4617) -> (-113.6903, 116.5257)
  line L374 (-113.6903, 116.5257) -> (-113.6903, 113.4617)
  line L375 (-113.6903, 113.4617) -> (-114.0854, 113.4617)
  line L376 (-114.0854, 113.4617) -> (-114.0854, 117.4617)
  line L377 (-114.0854, 117.4617) -> (-113.9948, 117.4617)
  line L378 (-113.9948, 117.4617) -> (-111.3551, 114.4334)
  line L379 (-111.3551, 114.4334) -> (-111.3551, 117.4617)
  line L380 (-111.3551, 117.4617) -> (-110.9405, 117.4617)
  line L381 (-115.0603, 113.4617) -> (-117.3535, 113.4617)
  line L382 (-117.3535, 113.4617) -> (-117.3535, 113.8536)
  line L383 (-117.3535, 113.8536) -> (-115.4587, 113.8536)
  line L384 (-115.4587, 113.8536) -> (-115.4587, 115.107)
  line L385 (-115.4587, 115.107) -> (-117.3373, 115.107)
  line L386 (-117.3373, 115.107) -> (-117.3373, 115.4989)
  line L387 (-117.3373, 115.4989) -> (-115.4587, 115.4989)
  line L388 (-115.4587, 115.4989) -> (-115.4587, 117.0698)
  line L389 (-115.4587, 117.0698) -> (-117.3373, 117.0698)
  line L390 (-117.3373, 117.0698) -> (-117.3373, 117.4617)
  line L391 (-117.3373, 117.4617) -> (-115.0603, 117.4617)
  line L392 (-115.0603, 117.4617) -> (-115.0603, 113.4617)
  line L393 (-119.1737, 116.7168) -> (-119.5138, 116.5127)
  spline S119 degree 2 poles (-119.5138, 116.5127) (-119.8733, 117.1734) (-120.3429, 117.1734) knots 0 0 0 1 1 1
  spline S120 degree 2 poles (-120.3429, 117.1734) (-120.5437, 117.1734) (-120.8968, 116.9856) (-121.0814, 116.6714) (-121.0814, 116.4933) knots 0 0 0 1 2 3 3 3
  spline S121 degree 2 poles (-121.0814, 116.4933) (-121.0814, 116.2925) (-120.9454, 116.1014) knots 0 0 0 1 1 1
  spline S122 degree 2 poles (-120.9454, 116.1014) (-120.7575, 115.8325) (-120.262, 115.4568) knots 0 0 0 1 1 1
  spline S123 degree 2 poles (-120.262, 115.4568) (-119.7599, 115.0811) (-119.6369, 114.9127) knots 0 0 0 1 1 1
  spline S124 degree 2 poles (-119.6369, 114.9127) (-119.4263, 114.6277) (-119.4263, 114.3006) knots 0 0 0 1 1 1
  spline S125 degree 2 poles (-119.4263, 114.3006) (-119.4263, 114.0382) (-119.6757, 113.6074) (-120.1292, 113.3613) (-120.3948, 113.3613) knots 0 0 0 1 2 3 3 3
  spline S126 degree 2 poles (-120.3948, 113.3613) (-120.6798, 113.3613) (-121.1688, 113.6431) (-121.4441, 114.0188) knots 0 0 0 1 2 2 2
  line L394 (-121.4441, 114.0188) -> (-121.117, 114.2649)
  spline S127 degree 2 poles (-121.117, 114.2649) (-120.8935, 113.967) (-120.5729, 113.7759) (-120.3883, 113.7759) knots 0 0 0 1 2 2 2
  spline S128 degree 2 poles (-120.3883, 113.7759) (-120.1454, 113.7759) (-119.8377, 114.0706) (-119.8377, 114.2844) knots 0 0 0 1 2 2 2
  spline S129 degree 2 poles (-119.8377, 114.2844) (-119.8377, 114.4139) (-119.9478, 114.6601) (-120.0903, 114.8026) knots 0 0 0 1 2 2 2
  spline S130 degree 2 poles (-120.0903, 114.8026) (-120.168, 114.8803) (-120.6085, 115.2042) knots 0 0 0 1 1 1
  spline S131 degree 2 poles (-120.6085, 115.2042) (-121.1267, 115.5864) (-121.5122, 116.1856) (-121.5122, 116.4868) knots 0 0 0 1 2 2 2
  spline S132 degree 2 poles (-121.5122, 116.4868) (-121.5122, 116.9208) (-120.8514, 117.5621) (-120.3786, 117.5621) knots 0 0 0 1 2 2 2
  spline S133 degree 2 poles (-120.3786, 117.5621) (-120.0158, 117.5621) (-119.4231, 117.1734) (-119.1737, 116.7168) knots 0 0 0 1 2 2 2
  line L395 (-122.3607, 113.4617) -> (-124.6539, 113.4617)
  line L396 (-124.6539, 113.4617) -> (-124.6539, 113.8536)
  line L397 (-124.6539, 113.8536) -> (-122.7591, 113.8536)
  line L398 (-122.7591, 113.8536) -> (-122.7591, 115.107)
  line L399 (-122.7591, 115.107) -> (-124.6377, 115.107)
  line L400 (-124.6377, 115.107) -> (-124.6377, 115.4989)
  line L401 (-124.6377, 115.4989) -> (-122.7591, 115.4989)
  line L402 (-122.7591, 115.4989) -> (-122.7591, 117.0698)
  line L403 (-122.7591, 117.0698) -> (-124.6377, 117.0698)
  line L404 (-124.6377, 117.0698) -> (-124.6377, 117.4617)
  line L405 (-124.6377, 117.4617) -> (-122.3607, 117.4617)
  line L406 (-122.3607, 117.4617) -> (-122.3607, 113.4617)
  line L407 (-125.347, 117.4617) -> (-125.347, 113.4617)
  line L408 (-125.347, 113.4617) -> (-125.4344, 113.4617)
  line L409 (-125.4344, 113.4617) -> (-128.0968, 116.5257)
  line L410 (-128.0968, 116.5257) -> (-128.0968, 113.4617)
  line L411 (-128.0968, 113.4617) -> (-128.4919, 113.4617)
  line L412 (-128.4919, 113.4617) -> (-128.4919, 117.4617)
  line L413 (-128.4919, 117.4617) -> (-128.4012, 117.4617)
  line L414 (-128.4012, 117.4617) -> (-125.7616, 114.4334)
  line L415 (-125.7616, 114.4334) -> (-125.7616, 117.4617)
  line L416 (-125.7616, 117.4617) -> (-125.347, 117.4617)
  line L417 (-129.4668, 117.4617) -> (-129.4668, 113.4617)
  line L418 (-129.4668, 113.4617) -> (-129.5543, 113.4617)
  line L419 (-129.5543, 113.4617) -> (-132.2166, 116.5257)
  line L420 (-132.2166, 116.5257) -> (-132.2166, 113.4617)
  line L421 (-132.2166, 113.4617) -> (-132.6118, 113.4617)
  line L422 (-132.6118, 113.4617) -> (-132.6118, 117.4617)
  line L423 (-132.6118, 117.4617) -> (-132.5211, 117.4617)
  line L424 (-132.5211, 117.4617) -> (-129.8814, 114.4334)
  line L425 (-129.8814, 114.4334) -> (-129.8814, 117.4617)
  line L426 (-129.8814, 117.4617) -> (-129.4668, 117.4617)
  line L427 (-134.8174, 115.7937) -> (-136.3105, 115.7937)
  line L428 (-136.3105, 115.7937) -> (-136.3105, 116.124)
  line L429 (-136.3105, 116.124) -> (-134.8174, 116.124)
  line L430 (-134.8174, 116.124) -> (-134.8174, 115.7937)
  line L431 (-139.0603, 113.4617) -> (-139.8474, 113.4617)
  line L432 (-139.8474, 113.4617) -> (-139.8474, 117.4617)
  line L433 (-139.8474, 117.4617) -> (-139.449, 117.4617)
  line L434 (-139.449, 117.4617) -> (-139.449, 113.8536)
  line L435 (-139.449, 113.8536) -> (-138.8207, 113.8536)
  line L436 (-138.8207, 113.8536) -> (-139.0603, 113.4617)
  spline S134 degree 2 poles (-143.2579, 115.2657) (-143.6628, 115.4666) (-144.0126, 115.9848) (-144.0126, 116.3119) knots 0 0 0 1 2 2 2
  spline S135 degree 2 poles (-144.0126, 116.3119) (-144.0126, 116.7751) (-143.7114, 117.1281) knots 0 0 0 1 1 1
  spline S136 degree 2 poles (-143.7114, 117.1281) (-143.3421, 117.5621) (-142.6522, 117.5621) knots 0 0 0 1 1 1
  spline S137 degree 2 poles (-142.6522, 117.5621) (-141.9915, 117.5621) (-141.3049, 116.8042) (-141.3049, 116.3443) knots 0 0 0 1 2 2 2
  spline S138 degree 2 poles (-141.3049, 116.3443) (-141.3049, 116.0107) (-141.6644, 115.473) (-142.0822, 115.2657) knots 0 0 0 1 2 2 2
  spline S139 degree 2 poles (-142.0822, 115.2657) (-141.7907, 115.1135) (-141.496, 114.6633) (-141.496, 114.4042) knots 0 0 0 1 2 2 2
  spline S140 degree 2 poles (-141.496, 114.4042) (-141.496, 114.1419) (-141.8101, 113.6463) (-142.3607, 113.3613) (-142.6814, 113.3613) knots 0 0 0 1 2 3 3 3
  spline S141 degree 2 poles (-142.6814, 113.3613) (-142.9923, 113.3613) (-143.5267, 113.6496) (-143.828, 114.1419) (-143.828, 114.4139) knots 0 0 0 1 2 3 3 3
  spline S142 degree 2 poles (-143.828, 114.4139) (-143.828, 114.686) (-143.5429, 115.1103) (-143.2579, 115.2657) knots 0 0 0 1 2 2 2